Autodesk Inventor part; units mm, degrees
(part 3 of 3)
  measures "d37" distance from line of point (0, 0) L36
  measures "d38" diameter of A27
  measures "d39" distance of L40.start A27.centre
  measures "d40" distance of L40.start L40.end
  measures "d41" radius of A28
  measures "d42" diameter of A29
  measures "d43" distance of L43.start A29.centre
  measures "d44" distance of L43.start L43.end
  measures "d45" radius of A30
  measures "d46" diameter of A31
  measures "d47" distance of L46.start A31.centre
  measures "d48" distance of L46.start L46.end
  measures "d49" radius of A32
  measures "d50" distance from line of point (0, 0) L38
  measures "d53" diameter of A33
  measures "d55" distance from line of L45 A33.centre
  measures "d60" distance of L49.end L50.end
  measures "d61" horizontal distance of point (-175, 0) point (-180, 21.55)
  measures "d62" horizontal distance of point (-110, 0) point (-115, 21.55)
  measures "d63" horizontal distance of point (-45, 0) point (-50, 21.55)
  measures "d64" distance from line of L38 point (15, 21.55)
  measures "d65" distance between parallel lines of L41 L67
  measures "d66" distance between parallel lines of L44 L71
  measures "d67" distance from line of A33.centre L75
  measures "d70" diameter of A34
  measures "d71" distance from line of L79 L76.end
  measures "d72" distance from line of L80 point (152.023, 0.85)
  measures "d73" distance from line of A27.centre L41
  measures "d74" distance between parallel lines of L41 L44
  measures "d75" distance from line of L44 A33.centre
  measures "d76" distance of A31.centre point (160, 0)
  measures "d77" distance from line of point (160, 0) L84
extrude "Extrusion2" cut sketch "Skizze4" against normal through all contours A12 | A13 | A14 | L18 A19 L19 A20 L20 A18 L21 A17 | A15 | A16 | L28 A25 L29 A26 L30 A24 L31 A23 | A21 | A22 | A28 A27 | A30 A29 | A32 A31 | A33 | L80 L79 L78 A34
extrude "Extrusion3" cut sketch "Skizze4" against normal blind 0.5 contours S0 L85 L86 L87 S1 S2 L88 L89 L90 S3 | S4 L91 L92 S5 S6 S7 S8 S9 S10 S11 S12 L93 L94 S13 S14 S15 S16 S17 S18 S19 | S20 S21 L95 L96 L97 S22 S23 S24 L98 S25 | L105 L106 L107 L108 L109 L110 | L111 L112 L113 L114 | L115 L116 L117 L118 | L119 S34 S35 S36 L120 L121 L122 S37 S38 S39 L123 L124 L125 L126 L127 S40 S41 S42 S43 S44 L128 L129 | L130 L131 L132 L133 | L134 L135 L136 L137 | S45 L138 L139 L140 L141 L142 L143 L144 L145 L146 L147 L148 S46 S47 S48 L149 L150 S49 | S50 L151 L152 S51 S52 S53 S54 S55 S56 S57 S58 L153 L154 S59 S60 S61 S62 S63 S64 S65 | L155 L156 L157 L158 L159 L160 L161 L162 L163 L164 L165 L166 L167 | L168 L169 L170 L171 | L172 L173 L174 L175 | S66 L176 L177 L178 L179 L180 L181 L182 L183 L184 L185 L186 S67 S68 S69 L187 L188 S70 | S71 S72 S73 S74 S75 L189 L190 S76 S77 S78 S79 S80 S81 L191 L192 S82 S83 | L193 L194 S84 S85 S86 L195 L196 L197 L198 L199 S87 S88 L200 | S89 S90 S91 L201 L202 S92 S93 S94 S95 L203 L204 S96 S97 | S100 L206 L207 S101 S102 S103 S104 S105 S106 S107 S108 S109 L208 L209 S110 S111 S112 S113 S114 S115 S116 S117 | L210 L211 L212 L213 L214 L215 L216 S118 S119 S120 L217 | S125 S126 S127 L221 L222 S128 S129 S130 S131 L223 L224 S132 S133 | L226 S136 S137 S138 L227 L228 L229 S139 S140 S141 L230 L231 L232 L233 L234 S142 S143 S144 S145 S146 L235 L236 | S147 S148 S149 S150 | S159 L237 L238 L239 L240 L241 L242 L243 L244 L245 L246 L247 S160 S161 S162 L248 L249 S163 | S164 S165 S166 L250 L251 S167 S168 S169 S170 L252 L253 S171 S172 | S175 S176 S177 S178 L255 L256 S179 S180 S181 S182 S183 S184 S185 S186 L257 L258 S187 S188 | S189 S190 S191 S192 | L259 L260 S201 S202 S203 L261 L262 L263 L264 L265 S204 S205 L266 | S206 L267 L268 L269 L270 L271 L272 L273 L274 L275 L276 L277 S207 S208 S209 L278 L279 S210 | L280 S211 S212 L281 L282 L283 L284 L285 S213 S214 S215 L286 | S216 S217 S218 S219 | L287 L288 L289 L290 | L291 L292 L293 L294 L295 L296 L297 L298 L299 L300 L301 L302 L303 | S228 S229 S230 S231 | S240 L304 L305 L306 L307 L308 L309 L310 L311 L312 L313 L314 S241 S242 S243 L315 L316 S244 | S245 S246 S247 S248 | L317 S257 S258 L318 L319 L320 L321 L322 S259 S260 S261 L323 | L324 L325 L326 L327 L328 L329 L330 L331 L332 L333 L334 L335 | L336 L337 L338 L339 L340 L341 L342 L343 L344 L345 L346 L347 L348 | S262 S263 S264 S265 | S274 L349 L350 L351 L352 L353 L354 L355 L356 L357 L358 L359 S275 S276 S277 L360 L361 S278 | S279 S280 S281 S282 | L362 S291 S292 L363 L364 L365 L366 L367 S293 S294 S295 L368 | L369 L370 L371 L372 L373 L374 L375 L376 L377 | L378 L379 L380 L381 L382 L383 L384 L385 L386 L387 L388 L389 L390 | S296 S297 S298 S299 | S308 L391 L392 L393 L394 L395 L396 L397 L398 L399 L400 L401 S309 S310 S311 L402 L403 S312 | S313 S314 S315 S316 | L404 S325 S326 L405 L406 L407 L408 L409 S327 S328 S329 L410 | L411 L412 L413 L414 L415 L416 L417 L418 L419 L420 | S330 S331 S332 L421 L422 L423 L424 L425 S333 S334 | S340 S341 S342 S343 | L429 L430 L431 L432 L433 L434 L435 L436 L437 L438 L439 L440 L441 | S352 S353 S354 L442 L443 S355 S356 S357 S358 L444 L445 S359 S360 | L447 S363 S364 L448 L449 L450 L451 L452 S365 S366 S367 L453 | L454 L455 L456 L457 L458 L459 L460 L461 L462 L463 L464 L465 | L466 S368 S369 S370 L467 L468 L469 S371 S372 S373 L470 L471 L472 L473 L474 S374 S375 S376 S377 S378 L475 L476 | S379 S380 S381 L477 L478 S382 S383 S384 S385 L479 L480 S386 S387 | L482 S390 S391 L483 L484 L485 L486 L487 S392 S393 S394 L488 | S395 S396 S397 L489 L490 S398 S399 S400 S401 L491 S402 S403 S404 S405 S406 L492 L493 L494 | S412 S413 S414 L496 L497 S415 S416 S417 S418 L498 L499 S419 S420 | L501 L502 S423 S424 S425 L503 L504 L505 L506 L507 S426 S427 L508 | S428 S429 S430 S431 S432 L509 L510 S433 S434 S435 S436 S437 S438 L511 L512 S439 S440 | L513 L514 L515 L516 L517 L518 L519 L520 | S441 L521 L522 S442 S443 S444 S445 S446 S447 S448 S449 L523 L524 S450 S451 S452 S453 S454 S455 S456 | S457 L525 L526 L527 L528 L529 L530 L531 L532 L533 L534 L535 S458 S459 S460 L536 L537 S461 | S462 S463 S464 S465 | S474 S475 L538 L539 L540 L541 L542 S476 S477
